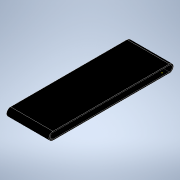
# Autodesk Inventor part: BELT
Saved by Autodesk Inventor 2021 (Build 250183000, 183)
## iProperties
Created: 2021-07-27
Part Number: BELT
Material: Generic
Document SubType Name: Modeling
Designer: HP
Density: 1 g/cm^3
Appearance: Anodized - Black
Author: HP
Autodesk Inventor part; units mm, degrees
ref_plane "YZ Plane" through (0, 0, 0) normal (1, 0, 0) x (0, 1, 0)
ref_plane "XZ Plane" through (0, 0, 0) normal (0, 1, 0) x (-1, 0, 0)
ref_plane "XY Plane" through (0, 0, 0) normal (0, 0, 1) x (1, 0, 0)
sketch "Sketch1" plane through (0, 0, 0) normal (1, 0, 0) x (0, 1, 0)
  arc A0 (-9.525, -17.4625) -> (9.525, -17.4625) centre (0, -17.4625) ccw
  line L0 (9.525, -17.4625) -> (9.525, 261.9375)
  arc A1 (9.525, 261.9375) -> (-9.525, 261.9375) centre (0, 261.9375) ccw
  line L1 (-9.525, 261.9375) -> (-9.525, -17.4625)
  arc A2 (-6.985, -17.4625) -> (6.985, -17.4625) centre (0, -17.4625) ccw
  arc A3 (6.985, 261.9375) -> (-6.985, 261.9375) centre (0, 261.9375) ccw
  line L2 (6.985, 261.9375) -> (6.985, -17.4625)
  line L3 (-6.985, -17.4625) -> (-6.985, 261.9375)
  point P0 (0, 0)
  dimension "d0" = 9.525
  dimension "d1" = 279.4
  dimension "d2" = 6.985
  dimension "d3" = 6.985
  constraints: 8 end point, 8 point on circle, 4 centre point, 2 coincident, 2 parallel, 2 vertical, 1 tangent
  measures "d0" radius of A0
  measures "d1" distance of L0.start L0.end
  measures "d2" radius of A2
  measures "d3" radius of A3
extrude "Extrusion1" add sketch "Sketch1" along normal blind 101.6
sketch "Sketch2" plane through (101.6, 0, 0) normal (1, 0, 0) x (0, 0, -1)
  point P0 (0, 0)
body "Solid1"
